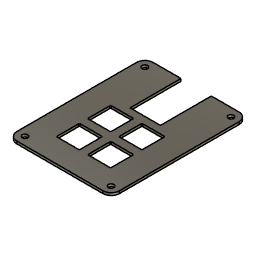
keyboard top v1 (Autodesk Fusion 360 design; units mm, degrees)
Autodesk Fusion 360 part; units mm, degrees
sketch "plate-2025-06-15T06_11_47.601Z" plane through (0, 0, 0) normal (0, 0, 1) x (1, 0, 0)
  line L0 (22.075, -40.625) -> (35.075, -40.625)
  line L1 (22.075, -54.625) -> (35.075, -54.625)
  line L2 (21.575, -41.125) -> (21.575, -54.125)
  line L3 (35.575, -41.125) -> (35.575, -54.125)
  arc A0 (22.075, -40.625) -> (21.575, -41.125) centre (22.075, -41.125) ccw
  arc A1 (35.575, -41.125) -> (35.075, -40.625) centre (35.075, -41.125) ccw
  arc A2 (21.575, -54.125) -> (22.075, -54.625) centre (22.075, -54.125) ccw
  arc A3 (35.075, -54.625) -> (35.575, -54.125) centre (35.075, -54.125) ccw
  line L4 (41.125, -40.625) -> (54.125, -40.625)
  line L5 (41.125, -54.625) -> (54.125, -54.625)
  line L6 (40.625, -41.125) -> (40.625, -54.125)
  line L7 (54.625, -41.125) -> (54.625, -54.125)
  arc A4 (41.125, -40.625) -> (40.625, -41.125) centre (41.125, -41.125) ccw
  arc A5 (54.625, -41.125) -> (54.125, -40.625) centre (54.125, -41.125) ccw
  arc A6 (40.625, -54.125) -> (41.125, -54.625) centre (41.125, -54.125) ccw
  arc A7 (54.125, -54.625) -> (54.625, -54.125) centre (54.125, -54.125) ccw
  line L8 (22.075, -59.675) -> (35.075, -59.675)
  line L9 (22.075, -73.675) -> (35.075, -73.675)
  line L10 (21.575, -60.175) -> (21.575, -73.175)
  line L11 (35.575, -60.175) -> (35.575, -73.175)
  arc A8 (22.075, -59.675) -> (21.575, -60.175) centre (22.075, -60.175) ccw
  arc A9 (35.575, -60.175) -> (35.075, -59.675) centre (35.075, -60.175) ccw
  arc A10 (21.575, -73.175) -> (22.075, -73.675) centre (22.075, -73.175) ccw
  arc A11 (35.075, -73.675) -> (35.575, -73.175) centre (35.075, -73.175) ccw
  line L12 (41.125, -59.675) -> (54.125, -59.675)
  line L13 (41.125, -73.675) -> (54.125, -73.675)
  line L14 (40.625, -60.175) -> (40.625, -73.175)
  line L15 (54.625, -60.175) -> (54.625, -73.175)
  arc A12 (41.125, -59.675) -> (40.625, -60.175) centre (41.125, -60.175) ccw
  arc A13 (54.625, -60.175) -> (54.125, -59.675) centre (54.125, -60.175) ccw
  arc A14 (40.625, -73.175) -> (41.125, -73.675) centre (41.125, -73.175) ccw
  arc A15 (54.125, -73.675) -> (54.625, -73.175) centre (54.125, -73.175) ccw
  line L16 (6.85, -88.072) -> (69.35, -88.072)
  line L17 (69.35, -88.072) -> (69.35, -5.072)
  line L18 (69.35, -5.072) -> (6.85, -5.072)
  line L19 (6.85, -5.072) -> (6.85, -88.072)
  circle A16 centre (11.85, -83.072) radius 1.7
  circle A17 centre (64.35, -83.072) radius 1.7
  circle A18 centre (11.85, -10.072) radius 1.7
  circle A19 centre (64.35, -10.072) radius 1.7
  line L20 (28.85, -5.072) -> (47.35, -5.072)
  line L21 (47.35, -5.072) -> (47.35, -36.072)
  line L22 (47.35, -36.072) -> (28.85, -36.072)
  line L23 (28.85, -36.072) -> (28.85, -5.072)
  dimension "d1" = 83
  dimension "d2" = 62.5
  dimension "d3" = 14.725
  dimension "d4" = 3.4
  dimension "d5" = 5
  dimension "d6" = 5
  dimension "d7" = 3.4
  dimension "d8" = 5
  dimension "d9" = 5
  dimension "d10" = 3.4
  dimension "d11" = 5
  dimension "d12" = 5
  dimension "d13" = 3.4
  dimension "d14" = 5
  dimension "d15" = 5
  dimension "d16" = 14.397
  dimension "d17" = 18.5
  dimension "d18" = 31
  dimension "d19" = 22
  constraint horizontal L16
  constraint vertical L17
  constraint horizontal L18
  constraint vertical L19
  constraint horizontal L20
  constraint vertical L21
  constraint horizontal L22
  constraint vertical L23
  constraint coincident L18 L20.start
  measures "d1" distance of L16 L18
  measures "d2" distance of L17 L19
  measures "d3" distance of L10 L19
  measures "d4" diameter of A16
  measures "d5" distance of L16 A16.centre
  measures "d6" distance of L19 A16.centre
  measures "d7" diameter of A17
  measures "d8" distance of L16 A17.centre
  measures "d9" distance of L17 A17.centre
  measures "d10" diameter of A18
  measures "d11" distance of L18 A18.centre
  measures "d12" distance of L19 A18.centre
  measures "d13" diameter of A19
  measures "d14" distance of L17 A19.centre
  measures "d15" distance of L18 A19.centre
  measures "d16" distance of L9 L16
  measures "d17" distance of L20.start L20.end
  measures "d18" distance of L20.start L22.end
  measures "d19" distance of L19 L23
extrude "Extrude1" add sketch "plate-2025-06-15T06_11_47.601Z" along normal blind 1.5 contours L16 L17 L18 L19 L21 L22 L23
fillet "Fillet1" radius 5 1 edges at (69.35, -88.072, 0.75)
fillet "Fillet2" radius 5 1 edges at (6.85, -88.072, 0.75)
fillet "Fillet3" radius 5 1 edges at (69.35, -5.072, 0.75)
fillet "Fillet4" radius 5 1 edges at (6.85, -5.072, 0.75)
sketch "Sketch2" plane through (0, 0, 0) normal (0, 0, -1) x (1, 0, 0)
  arc A0 (21.575, 41.125) -> (22.075, 40.625) centre (22.075, 41.125) ccw
  line L0 (21.575, 41.125) -> (21.575, 54.125)
  arc A1 (22.075, 54.625) -> (21.575, 54.125) centre (22.075, 54.125) ccw
  line L1 (22.075, 54.625) -> (35.075, 54.625)
  arc A2 (35.575, 54.125) -> (35.075, 54.625) centre (35.075, 54.125) ccw
  line L2 (35.575, 54.125) -> (35.575, 41.125)
  arc A3 (35.075, 40.625) -> (35.575, 41.125) centre (35.075, 41.125) ccw
  line L3 (35.075, 40.625) -> (22.075, 40.625)
  arc A4 (40.625, 60.175) -> (41.125, 59.675) centre (41.125, 60.175) ccw
  line L4 (40.625, 60.175) -> (40.625, 73.175)
  arc A5 (41.125, 73.675) -> (40.625, 73.175) centre (41.125, 73.175) ccw
  line L5 (41.125, 73.675) -> (54.125, 73.675)
  arc A6 (54.625, 73.175) -> (54.125, 73.675) centre (54.125, 73.175) ccw
  line L6 (54.625, 73.175) -> (54.625, 60.175)
  arc A7 (54.125, 59.675) -> (54.625, 60.175) centre (54.125, 60.175) ccw
  line L7 (54.125, 59.675) -> (41.125, 59.675)
  arc A8 (21.575, 60.175) -> (22.075, 59.675) centre (22.075, 60.175) ccw
  line L8 (21.575, 60.175) -> (21.575, 73.175)
  arc A9 (22.075, 73.675) -> (21.575, 73.175) centre (22.075, 73.175) ccw
  line L9 (22.075, 73.675) -> (35.075, 73.675)
  arc A10 (35.575, 73.175) -> (35.075, 73.675) centre (35.075, 73.175) ccw
  line L10 (35.575, 73.175) -> (35.575, 60.175)
  arc A11 (35.075, 59.675) -> (35.575, 60.175) centre (35.075, 60.175) ccw
  line L11 (35.075, 59.675) -> (22.075, 59.675)
  circle A12 centre (64.35, 83.072) radius 1.7
  circle A13 centre (64.35, 10.072) radius 1.7
  arc A14 (40.625, 41.125) -> (41.125, 40.625) centre (41.125, 41.125) ccw
  line L12 (40.625, 41.125) -> (40.625, 54.125)
  arc A15 (41.125, 54.625) -> (40.625, 54.125) centre (41.125, 54.125) ccw
  line L13 (41.125, 54.625) -> (54.125, 54.625)
  arc A16 (54.625, 54.125) -> (54.125, 54.625) centre (54.125, 54.125) ccw
  line L14 (54.625, 54.125) -> (54.625, 41.125)
  arc A17 (54.125, 40.625) -> (54.625, 41.125) centre (54.125, 41.125) ccw
  line L15 (54.125, 40.625) -> (41.125, 40.625)
  circle A18 centre (11.85, 83.072) radius 1.7
  circle A19 centre (11.85, 10.072) radius 1.7
  arc A20 (6.85, 10.072) -> (11.85, 5.072) centre (11.85, 10.072) ccw
  line L16 (11.85, 5.072) -> (28.85, 5.072)
  line L17 (28.85, 5.072) -> (28.85, 36.072)
  line L18 (28.85, 36.072) -> (47.35, 36.072)
  line L19 (47.35, 36.072) -> (47.35, 5.072)
  line L20 (47.35, 5.072) -> (64.35, 5.072)
  arc A21 (64.35, 5.072) -> (69.35, 10.072) centre (64.35, 10.072) ccw
  line L21 (69.35, 10.072) -> (69.35, 83.072)
  arc A22 (69.35, 83.072) -> (64.35, 88.072) centre (64.35, 83.072) ccw
  line L22 (64.35, 88.072) -> (11.85, 88.072)
  arc A23 (11.85, 88.072) -> (6.85, 83.072) centre (11.85, 83.072) ccw
  line L23 (6.85, 83.072) -> (6.85, 10.072)
  line L24 (22, 78) -> (54, 78) construction
  line L25 (54, 78) -> (54, 84) construction
  line L26 (54, 84) -> (22, 84) construction
  line L27 (22, 84) -> (22, 78) construction
  dimension "d30" = 1
  text T0 "Jessica's Keyboard" font "Arial" height 1 align centre middle in box 32 x 6 at (22, 78) x (1, 0) y (0, 1) spacing 1
extrude "Extrude2" cut sketch "Sketch2" against normal blind 0.2 text T0
